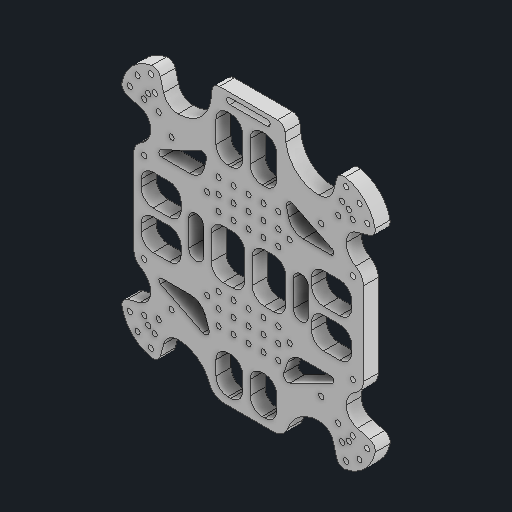
# Autodesk Inventor part: top
Saved by Autodesk Inventor 2023 (Build 270158000, 158)
## iProperties
Created: 2022-06-01
Part Number: top
Material: Generic
Document SubType Name: Modeling
Designer: vibhu
Density: 1 g/cm^3
Appearance: Default
Author: vibhu
Autodesk Inventor part; units mm, degrees
ref_plane "YZ Plane" through (0, 0, 0) normal (1, 0, 0) x (0, 1, 0)
ref_plane "XZ Plane" through (0, 0, 0) normal (0, 1, 0) x (-1, 0, 0)
ref_plane "Work Plane1" through (0, 0, 0) normal (0, 0, 1) x (1, 0, 0)
sketch "Sketch1" plane through (0, 0, 0) normal (0, 0, 1) x (1, 0, 0)
  arc A0 (58.1462, -72.4732) -> (48.4869, -65.0614) centre (48.4869, -75.0614) ccw projected
  line L0 (60.3557, -80.7192) -> (58.1462, -72.4732) projected
  arc A1 (60.3557, -80.7192) -> (66.1208, -84.3368) centre (65.1853, -79.4251) ccw projected
  arc A2 (66.1208, -84.3368) -> (86.0018, -64.4558) centre (61.4433, -59.7783) ccw projected
  arc A3 (86.0018, -64.4558) -> (82.3842, -58.6907) centre (81.0901, -63.5203) ccw projected
  line L1 (74.1382, -56.4812) -> (82.3842, -58.6907) projected
  arc A4 (66.7264, -46.8219) -> (74.1382, -56.4812) centre (76.7264, -46.8219) ccw projected
  circle A5 centre (61.4433, -59.7783) radius 1.75 projected
  circle A6 centre (68.5144, -66.8494) radius 1.75 projected
  circle A7 centre (64.0315, -69.4376) radius 1.75 projected
  circle A8 centre (71.1025, -62.3665) radius 1.75 projected
  circle A9 centre (80.7618, -64.9547) radius 1.75 projected
  circle A10 centre (75.5854, -73.9204) radius 1.75 projected
  circle A11 centre (66.6197, -79.0968) radius 1.75 projected
  line L2 (-55.2596, -72.4732) -> (-57.4691, -80.7192) projected
  arc A12 (-63.2342, -84.3368) -> (-57.4691, -80.7192) centre (-62.2987, -79.4251) ccw projected
  arc A13 (-83.1152, -64.4558) -> (-63.2342, -84.3368) centre (-58.5567, -59.7783) ccw projected
  arc A14 (-79.4976, -58.6907) -> (-83.1152, -64.4558) centre (-78.2035, -63.5203) ccw projected
  line L3 (-79.4976, -58.6907) -> (-71.2516, -56.4812) projected
  arc A15 (-71.2516, -56.4812) -> (-63.8398, -46.8219) centre (-73.8398, -46.8219) ccw projected
  arc A16 (-45.6003, -65.0614) -> (-55.2596, -72.4732) centre (-45.6003, -75.0614) ccw projected
  circle A17 centre (-61.1449, -69.4376) radius 1.75 projected
  circle A18 centre (-58.5567, -59.7783) radius 1.75 projected
  circle A19 centre (-65.6278, -66.8494) radius 1.75 projected
  circle A20 centre (-68.216, -62.3665) radius 1.75 projected
  circle A21 centre (-77.8752, -64.9547) radius 1.75 projected
  circle A22 centre (-72.6989, -73.9204) radius 1.75 projected
  circle A23 centre (-63.7331, -79.0968) radius 1.75 projected
  arc A24 (-63.8398, 47.2653) -> (-71.2516, 56.9246) centre (-73.8398, 47.2653) ccw projected
  line L4 (-71.2516, 56.9246) -> (-79.4976, 59.1341) projected
  arc A25 (-83.1152, 64.8992) -> (-79.4976, 59.1341) centre (-78.2035, 63.9637) ccw projected
  circle A26 centre (-77.8752, 65.3981) radius 1.75 projected
  arc A27 (-63.2342, 84.7802) -> (-83.1152, 64.8992) centre (-58.5567, 60.2217) ccw projected
  circle A28 centre (-68.216, 62.8099) radius 1.75 projected
  circle A29 centre (-58.5567, 60.2217) radius 1.75 projected
  circle A30 centre (-65.6278, 67.2928) radius 1.75 projected
  circle A31 centre (-61.1449, 69.881) radius 1.75 projected
  circle A32 centre (-72.6989, 74.3638) radius 1.75 projected
  circle A33 centre (-63.7331, 79.5402) radius 1.75 projected
  arc A34 (-57.4691, 81.1626) -> (-63.2342, 84.7802) centre (-62.2987, 79.8685) ccw projected
  line L5 (-57.4691, 81.1626) -> (-55.2596, 72.9166) projected
  arc A35 (-55.2596, 72.9166) -> (-45.6003, 65.5048) centre (-45.6003, 75.5048) ccw projected
  line L6 (13.9433, 88.2217) -> (-11.0567, 88.2217) projected
  arc A36 (13.9433, 88.2217) -> (13.9433, 92.2217) centre (13.9433, 90.2217) ccw projected
  line L7 (-11.0567, 92.2217) -> (13.9433, 92.2217) projected
  arc A37 (-11.0567, 92.2217) -> (-11.0567, 88.2217) centre (-11.0567, 90.2217) ccw projected
  line L8 (20.8532, 95.2217) -> (-17.9667, 95.2217) projected
  circle A38 centre (-18.5567, 80.2217) radius 1.75 construction
  circle A39 centre (-18.5567, 60.2217) radius 1.75 construction
  circle A40 centre (21.4433, 60.2217) radius 1.75 construction
  circle A41 centre (21.4433, 80.2217) radius 1.75 construction
  circle A42 centre (1.4433, 80.2217) radius 1.75 construction
  circle A43 centre (1.4433, 60.2217) radius 1.75 construction
  arc A44 (48.4869, 65.5048) -> (58.1462, 72.9166) centre (48.4869, 75.5048) ccw projected
  line L9 (58.1462, 72.9166) -> (60.3557, 81.1626) projected
  arc A45 (66.1208, 84.7802) -> (60.3557, 81.1626) centre (65.1853, 79.8685) ccw projected
  arc A46 (86.0018, 64.8992) -> (66.1208, 84.7802) centre (61.4433, 60.2217) ccw projected
  arc A47 (82.3842, 59.1341) -> (86.0018, 64.8992) centre (81.0901, 63.9637) ccw projected
  line L10 (82.3842, 59.1341) -> (74.1382, 56.9246) projected
  arc A48 (74.1382, 56.9246) -> (66.7264, 47.2653) centre (76.7264, 47.2653) ccw projected
  circle A49 centre (61.4433, 60.2217) radius 1.75 projected
  circle A50 centre (68.5144, 67.2928) radius 1.75 projected
  circle A51 centre (71.1025, 62.8099) radius 1.75 projected
  circle A52 centre (64.0315, 69.881) radius 1.75 projected
  circle A53 centre (66.6197, 79.5402) radius 1.75 projected
  circle A54 centre (75.5854, 74.3638) radius 1.75 projected
  circle A55 centre (80.7618, 65.3981) radius 1.75 projected
  circle A56 centre (71.4433, -19.7783) radius 1.75 construction
  circle A57 centre (51.4433, -19.7783) radius 1.75 construction
  circle A58 centre (51.4433, 20.2217) radius 1.75 construction
  circle A59 centre (61.4433, 20.2217) radius 1.75 construction
  circle A60 centre (-48.5567, 20.2217) radius 1.75 construction
  circle A61 centre (-68.5567, 20.2217) radius 1.75 construction
  circle A62 centre (-68.5567, -19.7783) radius 1.75 construction
  circle A63 centre (-48.5567, -19.7783) radius 1.75 construction
  circle A64 centre (-68.5567, 0.2217) radius 1.75 construction
  circle A65 centre (-48.5567, 0.2217) radius 1.75 construction
  circle A66 centre (-18.5567, -9.7783) radius 1.75 construction
  circle A67 centre (-18.5567, 10.2217) radius 1.75 construction
  circle A68 centre (21.4433, 10.2217) radius 1.75 construction
  circle A69 centre (21.4433, -9.7783) radius 1.75 construction
  circle A70 centre (1.4433, -9.7783) radius 1.75 construction
  circle A71 centre (1.4433, 10.2217) radius 1.75 construction
  circle A72 centre (-26.0567, -29.7783) radius 1.75 projected
  circle A73 centre (-26.0567, 30.2217) radius 1.75 projected
  circle A74 centre (28.9433, -29.7783) radius 1.75 projected
  circle A75 centre (28.9433, 30.2217) radius 1.75 projected
  circle A76 centre (-18.5567, -59.7783) radius 1.75 construction
  circle A77 centre (21.4433, -59.7783) radius 1.75 construction
  circle A78 centre (1.4433, -59.7783) radius 1.75 construction
  circle A79 centre (1.4433, -79.7783) radius 1.75 construction
  circle A80 centre (21.4433, -79.7783) radius 1.75 construction
  circle A81 centre (-18.5567, -79.7783) radius 1.75 construction
  arc A82 (-70.1082, 36.6881) -> (-63.8398, 47.2653) centre (-75.8979, 47.2653) ccw projected
  arc A83 (-70.1082, 36.6881) -> (-75.3067, 27.9162) centre (-65.3067, 27.9162) ccw projected
  line L11 (-75.3067, 27.9162) -> (-75.3067, -27.4729) projected
  arc A84 (-75.3067, -27.4729) -> (-70.1082, -36.2447) centre (-65.3067, -27.4729) ccw projected
  arc A85 (-63.8398, -46.8219) -> (-70.1082, -36.2447) centre (-75.8979, -46.8219) ccw projected
  arc A86 (-24.7861, -79.8307) -> (-45.6003, -65.0614) centre (-45.6003, -87.1128) ccw projected
  arc A87 (-24.7861, -79.8307) -> (-15.3471, -86.5283) centre (-15.3471, -76.5283) ccw projected
  line L12 (-15.3471, -86.5283) -> (18.2337, -86.5283) projected
  arc A88 (18.2337, -86.5283) -> (27.6726, -79.8307) centre (18.2337, -76.5283) ccw projected
  arc A89 (48.4869, -65.0614) -> (27.6726, -79.8307) centre (48.4869, -87.1128) ccw projected
  arc A90 (72.9948, -36.2447) -> (66.7264, -46.8219) centre (78.7845, -46.8219) ccw projected
  arc A91 (72.9948, -36.2447) -> (78.1933, -27.4729) centre (68.1933, -27.4729) ccw projected
  line L13 (78.1933, -27.4729) -> (78.1933, 27.9162) projected
  arc A92 (78.1933, 27.9162) -> (72.9948, 36.6881) centre (68.1933, 27.9162) ccw projected
  arc A93 (66.7264, 47.2653) -> (72.9948, 36.6881) centre (78.7845, 47.2653) ccw projected
  arc A94 (26.4433, 85.2217) -> (48.4869, 65.5048) centre (48.4869, 87.6857) ccw projected
  line L14 (26.4433, 85.2217) -> (25.8223, 90.7771) projected
  arc A95 (25.8223, 90.7771) -> (20.8532, 95.2217) centre (20.8532, 90.2217) ccw projected
  arc A96 (-17.9667, 95.2217) -> (-22.9357, 90.7771) centre (-17.9667, 90.2217) ccw projected
  line L15 (-22.9357, 90.7771) -> (-23.5567, 85.2217) projected
  arc A97 (-45.6003, 65.5048) -> (-23.5567, 85.2217) centre (-45.6003, 87.6857) ccw projected
  circle A98 centre (-68.3067, 30.2217) radius 1.75 projected
  circle A99 centre (-68.3067, -29.7783) radius 1.75 projected
  circle A100 centre (71.1933, -29.7783) radius 1.75 projected
  circle A101 centre (71.1933, 30.2217) radius 1.75 projected
  arc A102 (-28.5567, 9.0414) -> (-38.5567, 9.0414) centre (-33.5567, 9.0414) ccw projected
  line L16 (-38.5567, -8.598) -> (-38.5567, 9.0414) projected
  arc A103 (-38.5567, -8.598) -> (-28.5567, -8.598) centre (-33.5567, -8.598) ccw projected
  line L17 (-28.5567, 9.0414) -> (-28.5567, -8.598) projected
  line L18 (31.4433, -8.598) -> (31.4433, 9.0414) projected
  arc A104 (41.4433, 9.0414) -> (31.4433, 9.0414) centre (36.4433, 9.0414) ccw projected
  line L19 (41.4433, 9.0414) -> (41.4433, -8.598) projected
  arc A105 (31.4433, -8.598) -> (41.4433, -8.598) centre (36.4433, -8.598) ccw projected
  line L20 (1.4433, 104.693) -> (1.4433, -135.8367) construction
  circle A106 centre (-18.5567, 22.451) radius 1.75
  line L21 (1.4433, -94.5531) -> (25.8223, -94.5531) construction
  circle A107 centre (-18.5567, 32.451) radius 1.75
  circle A108 centre (-18.5567, 42.451) radius 1.75
  circle A109 centre (-8.5567, 22.451) radius 1.75
  circle A110 centre (-8.5567, 32.451) radius 1.75
  circle A111 centre (-8.5567, 42.451) radius 1.75
  circle A112 centre (1.4433, 22.451) radius 1.75
  circle A113 centre (1.4433, 32.451) radius 1.75
  circle A114 centre (1.4433, 42.451) radius 1.75
  circle A115 centre (11.4433, 22.451) radius 1.75
  circle A116 centre (11.4433, 32.451) radius 1.75
  circle A117 centre (11.4433, 42.451) radius 1.75
  circle A118 centre (21.4433, 22.451) radius 1.75
  circle A119 centre (21.4433, 32.451) radius 1.75
  circle A120 centre (21.4433, 42.451) radius 1.75
  line L22 (-3.5567, 35.8119) -> (-34.2609, 35.8119) construction
  line L23 (-36.5279, 29.0902) -> (-8, 29.0902) construction
  line L24 (-15.4957, 35.8119) -> (-15.4957, 29.0902) construction
  circle A121 centre (-18.5567, -23.7293) radius 1.75
  circle A122 centre (-18.5567, -33.7293) radius 1.75
  circle A123 centre (-18.5567, -43.7293) radius 1.75
  circle A124 centre (-8.5567, -23.7293) radius 1.75
  circle A125 centre (-8.5567, -33.7293) radius 1.75
  circle A126 centre (-8.5567, -43.7293) radius 1.75
  circle A127 centre (1.4433, -23.7293) radius 1.75
  circle A128 centre (1.4433, -33.7293) radius 1.75
  circle A129 centre (1.4433, -43.7293) radius 1.75
  circle A130 centre (11.4433, -23.7293) radius 1.75
  circle A131 centre (11.4433, -33.7293) radius 1.75
  circle A132 centre (11.4433, -43.7293) radius 1.75
  circle A133 centre (21.4433, -23.7293) radius 1.75
  circle A134 centre (21.4433, -33.7293) radius 1.75
  circle A135 centre (21.4433, -43.7293) radius 1.75
  line L25 (-6.5567, -30.3685) -> (-35.0846, -30.3685) construction
  line L26 (-35.7042, -37.0902) -> (-5, -37.0902) construction
  line L27 (-15.1289, -30.3685) -> (-15.1289, -37.0902) construction
  point P0 (0, 0)
  point P1 (-75.3067, 0.2217)
  point P2 (-15.4957, 32.451)
  point P3 (-15.1289, -33.7293)
  dimension "d6" = 3.5
  dimension "d9" = 10
  dimension "d12" = 10
  dimension "d17" = 10
  dimension "d20" = 10
  constraints: 30 centre point, 12 end point, 6 point on line, 5 horizontal, 3 midpoint, 3 vertical, 2 horizontal alignment, 2 perpendicular, 2 vertical alignment, 1 equal radius, 60 other
  measures "d6" diameter of A106
  measures "d9" distance of A106.centre A107.centre
  measures "d12" distance of A106.centre A109.centre
  measures "d17" distance of A121.centre A122.centre
  measures "d20" distance of A121.centre A124.centre
extrude "Extrusion1" add sketch "Sketch1" along normal blind 10
sketch "Sketch2" plane through (0, 0, 10) normal (0, 0, 1) x (1, 0, 0)
  circle A0 centre (-18.5567, -59.7783) radius 1.75 construction
  circle A1 centre (-18.5567, -79.7783) radius 1.75 construction
  circle A2 centre (21.4433, -79.7783) radius 1.75 construction
  circle A3 centre (21.4433, -59.7783) radius 1.75 construction
  circle A4 centre (51.4433, -19.7783) radius 1.75 construction
  circle A5 centre (71.4433, -19.7783) radius 1.75 construction
  circle A6 centre (51.4433, 20.2217) radius 1.75 construction
  circle A7 centre (-68.5567, 20.2217) radius 1.75 construction
  circle A8 centre (-48.5567, 20.2217) radius 1.75 construction
  circle A9 centre (-68.5567, -19.7783) radius 1.75 construction
  circle A10 centre (-48.5567, -19.7783) radius 1.75 construction
  circle A11 centre (-18.5567, 60.2217) radius 1.75 construction
  circle A12 centre (21.4433, 60.2217) radius 1.75 construction
  circle A13 centre (21.4433, 80.2217) radius 1.75 construction
  circle A14 centre (-18.5567, 80.2217) radius 1.75 construction
  circle A15 centre (-18.5567, -9.7783) radius 1.75 construction
  circle A16 centre (21.4433, -9.7783) radius 1.75 construction
  circle A17 centre (21.4433, 10.2217) radius 1.75 construction
  circle A18 centre (-18.5567, 10.2217) radius 1.75 construction
  line L0 (-70.3067, 23.4717) -> (-43.5567, 23.4717)
  line L1 (-43.5567, 23.4717) -> (-43.5567, -23.0283)
  line L2 (-43.5567, -23.0283) -> (-70.3067, -23.0283)
  line L3 (-70.3067, -23.0283) -> (-70.3067, 23.4717)
  line L4 (-75.3067, 27.9162) -> (-75.3067, -27.4729) projected
  circle A19 centre (-68.3067, 30.2217) radius 1.75 projected
  line L5 (-38.5567, -8.598) -> (-38.5567, 9.0414) projected
  line L6 (-70.3067, 2.7217) -> (-43.5567, 2.7217)
  line L7 (-43.5567, 2.7217) -> (-43.5567, -2.2783)
  line L8 (-43.5567, -2.2783) -> (-70.3067, -2.2783)
  line L9 (-70.3067, -2.2783) -> (-70.3067, 2.7217)
  line L10 (-23.5567, 15.701) -> (26.4433, 15.701)
  line L11 (26.4433, 15.701) -> (26.4433, -16.9793)
  line L12 (26.4433, -16.9793) -> (-23.5567, -16.9793)
  line L13 (-23.5567, -16.9793) -> (-23.5567, 15.701)
  line L14 (-28.5567, 9.0414) -> (-28.5567, -8.598) projected
  line L15 (31.4433, -8.598) -> (31.4433, 9.0414) projected
  circle A20 centre (-18.5567, 22.451) radius 1.75 construction
  circle A21 centre (-18.5567, -23.7293) radius 1.75 construction
  line L16 (-1.0567, 15.701) -> (3.9433, 15.701)
  line L17 (3.9433, 15.701) -> (3.9433, -16.9793)
  line L18 (3.9433, -16.9793) -> (-1.0567, -16.9793)
  line L19 (-1.0567, -16.9793) -> (-1.0567, 15.701)
  line L20 (0, 120.2032) -> (0, -113.5378) construction
  line L21 (-20.3067, 83.2217) -> (20.3067, 83.2217)
  line L22 (20.3067, 83.2217) -> (20.3067, 52.451)
  line L23 (20.3067, 52.451) -> (-20.3067, 52.451)
  line L24 (-20.3067, 52.451) -> (-20.3067, 83.2217)
  line L25 (-2.5, 83.2217) -> (2.5, 83.2217)
  line L26 (2.5, 83.2217) -> (2.5, 52.451)
  line L27 (2.5, 52.451) -> (-2.5, 52.451)
  line L28 (-2.5, 52.451) -> (-2.5, 83.2217)
  line L29 (13.9433, 88.2217) -> (-11.0567, 88.2217) projected
  circle A22 centre (-18.5567, 42.451) radius 1.75 projected
  line L30 (0, 0) -> (110.9609, 0) construction
  circle A23 centre (68.5567, 20.2217) radius 1.75 construction
  circle A24 centre (48.5567, 20.2217) radius 1.75 construction
  circle A25 centre (68.5567, -19.7783) radius 1.75 construction
  circle A26 centre (48.5567, -19.7783) radius 1.75 construction
  line L31 (70.3067, 23.4717) -> (43.5567, 23.4717)
  line L32 (43.5567, 23.4717) -> (43.5567, -23.0283)
  line L33 (43.5567, -23.0283) -> (70.3067, -23.0283)
  line L34 (70.3067, -23.0283) -> (70.3067, 23.4717)
  line L35 (70.3067, 2.7217) -> (43.5567, 2.7217)
  line L36 (43.5567, 2.7217) -> (43.5567, -2.2783)
  line L37 (43.5567, -2.2783) -> (70.3067, -2.2783)
  line L38 (70.3067, -2.2783) -> (70.3067, 2.7217)
  line L39 (-20.3067, -56.0283) -> (20.3067, -56.0283)
  line L40 (20.3067, -56.0283) -> (20.3067, -81.5283)
  line L41 (20.3067, -81.5283) -> (-20.3067, -81.5283)
  line L42 (-20.3067, -81.5283) -> (-20.3067, -56.0283)
  line L43 (-2.5, -56.0283) -> (2.5, -56.0283)
  line L44 (2.5, -56.0283) -> (2.5, -81.5283)
  line L45 (2.5, -81.5283) -> (-2.5, -81.5283)
  line L46 (-2.5, -81.5283) -> (-2.5, -56.0283)
  line L47 (-15.3471, -86.5283) -> (18.2337, -86.5283) projected
  point P0 (-38.5567, 0.2217)
  point P1 (-43.5567, 0.2217)
  point P2 (-43.5567, 0.2217)
  point P3 (1.4433, 15.701)
  point P4 (1.4433, 15.701)
  point P5 (0, 83.2217)
  point P6 (0, 83.2217)
  point P7 (43.5567, 0.2217)
  point P8 (43.5567, 0.2217)
  point P9 (0, -56.0283)
  point P10 (0, -56.0283)
  point P11 (-43.5567, -2.2783)
  point P12 (-70.3067, -2.2783)
  point P13 (-70.3067, 2.7217)
  point P14 (-43.5567, 2.7217)
  point P15 (-1.0567, 15.701)
  point P16 (43.5567, 2.7217)
  point P17 (70.3067, 2.7217)
  point P18 (70.3067, -2.2783)
  point P19 (43.5567, -2.2783)
  dimension "d25" = 5
  dimension "d27" = 5
  dimension "d28" = 5
  dimension "d29" = 5
  dimension "d30" = 5
  dimension "d31" = 5
  dimension "d33" = 5
  dimension "d34" = 5
  dimension "d35" = 5
  dimension "d36" = 5
  dimension "d37" = 10
  dimension "d38" = 5
  dimension "d40" = 5
  dimension "d41" = 5
  dimension "d42" = 2
  constraints: 84 end point, 16 parallel, 14 symmetric about line, 9 horizontal, 9 midpoint, 8 collinear, 8 perpendicular, 4 centre point, 4 coincident, 3 point on line, 2 tangent, 1 horizontal alignment, 1 vertical, 4 other
  measures "d25" distance between parallel lines of L4 L3
  measures "d27" distance edge to line of A19 L0
  measures "d28" distance between parallel lines of L5 L1
  measures "d29" distance between parallel lines of L8 L6
  measures "d30" distance between parallel lines of L13 L14
  measures "d31" distance between parallel lines of L15 L11
  measures "d33" distance edge to line of A20 L10
  measures "d34" distance edge to line of A21 L12
  measures "d35" distance between parallel lines of L17 L19
  measures "d36" distance between parallel lines of L21 L29
  measures "d37" distance from line of A22.centre L23
  measures "d38" distance between parallel lines of L26 L28
  measures "d40" distance between parallel lines of L44 L46
  measures "d41" distance between parallel lines of L41 L47
  measures "d42" distance edge to line of A0 L39
extrude "Extrusion2" cut sketch "Sketch2" against normal up to surface (10 mm away) contours L0 L1 L6 L3 | L8 L1 L2 L3 | L10 L19 L12 L13 | L10 L11 L12 L17 | L21 L28 L23 L24 | L21 L22 L23 L26 | L34 L35 L32 L31 | L34 L33 L32 L37 | L39 L46 L41 L42 | L39 L40 L41 L44
fillet "Fillet1" radius 8 40 edges at (-43.5567, -23.0283, 5) (-43.5567, -2.2783, 5) (-43.5567, 23.4717, 5) (-43.5567, 2.7217, 5) (-70.3067, 23.4717, 5) (-70.3067, 2.7217, 5) (-70.3067, -2.2783, 5) (-70.3067, -23.0283, 5) (-20.3067, -56.0283, 5) (-2.5, -56.0283, 5) (2.5, -56.0283, 5) (20.3067, -56.0283, 5) (20.3067, -81.5283, 5) (2.5, -81.5283, 5) (-2.5, -81.5283, 5) (-20.3067, -81.5283, 5) (-1.0567, 15.701, 5) (-23.5567, 15.701, 5) (-23.5567, -16.9793, 5) (-1.0567, -16.9793, 5) (3.9433, -16.9793, 5) (3.9433, 15.701, 5) (26.4433, 15.701, 5) (26.4433, -16.9793, 5) (70.3067, 23.4717, 5) (70.3067, 2.7217, 5) (70.3067, -2.2783, 5) (70.3067, -23.0283, 5) (43.5567, -23.0283, 5) (43.5567, -2.2783, 5) (43.5567, 2.7217, 5) (43.5567, 23.4717, 5) (-2.5, 52.451, 5) (2.5, 52.451, 5) (2.5, 83.2217, 5) (-2.5, 83.2217, 5) (-20.3067, 83.2217, 5) (-20.3067, 52.451, 5) (20.3067, 83.2217, 5) (20.3067, 52.451, 5)
sketch "Sketch3" plane through (0, 0, 10) normal (0, 0, 1) x (1, 0, 0)
  line L0 (-50, 50) -> (50, 50) construction
  line L1 (50, 50) -> (50, -50) construction
  line L2 (50, -50) -> (-50, -50) construction
  line L3 (-50, -50) -> (-50, 50) construction
  line L4 (-50, 50) -> (50, -50) construction
  line L5 (50, 50) -> (-50, -50) construction
  circle A0 centre (-50, 50) radius 1.75
  circle A1 centre (50, 50) radius 1.75
  circle A2 centre (50, -50) radius 1.75
  circle A3 centre (-50, -50) radius 1.75
  point P0 (0, 0)
  dimension "d46" = 100
  dimension "d47" = 100
  dimension "d48" = 3.5
  constraints: 12 end point, 4 centre point, 4 coincident, 3 equal radius, 2 midpoint, 2 parallel, 1 horizontal, 1 perpendicular
  measures "d46" distance of L1.end L2.end
  measures "d47" distance of L0.end L1.end
  measures "d48" diameter of A0
extrude "Extrusion3" cut sketch "Sketch3" against normal up to surface (10 mm away)
sketch "Sketch4" plane through (0, 0, 0) normal (0, 0, -1) x (-1, 0, 0)
  circle A0 centre (-21.4433, 42.451) radius 1.75 construction
  circle A1 centre (-21.4433, 42.451) radius 3.25
  circle A2 centre (-21.4433, -23.7293) radius 1.75 construction
  circle A3 centre (-21.4433, -23.7293) radius 3.25
  line L0 (0, 0) -> (22.8644, 0) construction
  line L1 (22.8644, 0) -> (0, 0)
  line L2 (0, 16.9905) -> (0, 0) construction
  circle A4 centre (-11.4433, -23.7293) radius 3.25
  circle A5 centre (-1.4433, -23.7293) radius 3.25
  circle A6 centre (8.5567, -23.7293) radius 3.25
  circle A7 centre (18.5567, -23.7293) radius 3.25
  circle A8 centre (-21.4433, -33.7293) radius 3.25
  circle A9 centre (-11.4433, -33.7293) radius 3.25
  circle A10 centre (-1.4433, -33.7293) radius 3.25
  circle A11 centre (8.5567, -33.7293) radius 3.25
  circle A12 centre (18.5567, -33.7293) radius 3.25
  circle A13 centre (-21.4433, -43.7293) radius 3.25
  circle A14 centre (-11.4433, -43.7293) radius 3.25
  circle A15 centre (-1.4433, -43.7293) radius 3.25
  circle A16 centre (8.5567, -43.7293) radius 3.25
  circle A17 centre (18.5567, -43.7293) radius 3.25
  circle A18 centre (-11.4433, 42.451) radius 3.25
  circle A19 centre (-1.4433, 42.451) radius 3.25
  circle A20 centre (8.5567, 42.451) radius 3.25
  circle A21 centre (18.5567, 42.451) radius 3.25
  circle A22 centre (-21.4433, 32.451) radius 3.25
  circle A23 centre (-11.4433, 32.451) radius 3.25
  circle A24 centre (-1.4433, 32.451) radius 3.25
  circle A25 centre (8.5567, 32.451) radius 3.25
  circle A26 centre (18.5567, 32.451) radius 3.25
  circle A27 centre (-21.4433, 22.451) radius 3.25
  circle A28 centre (-11.4433, 22.451) radius 3.25
  circle A29 centre (-1.4433, 22.451) radius 3.25
  circle A30 centre (8.5567, 22.451) radius 3.25
  circle A31 centre (18.5567, 22.451) radius 3.25
  dimension "d51" = 6.5
  dimension "d52" = 6.5
  dimension "d60" = 10
  dimension "d63" = 10
  dimension "d68" = 10
  dimension "d71" = 10
  constraints: 30 centre point, 6 end point, 3 horizontal, 2 coincident, 2 vertical, 1 collinear, 1 perpendicular, 56 other
  measures "d51" diameter of A1
  measures "d52" diameter of A3
  measures "d60" distance of A3.centre A4.centre
  measures "d63" distance of A3.centre A8.centre
  measures "d68" distance of A1.centre A18.centre
  measures "d71" distance of A1.centre A22.centre
extrude "Extrusion4" cut sketch "Sketch4" against normal blind 3
sketch "Sketch5" plane through (0, 0, 10) normal (0, 0, 1) x (1, 0, 0)
  line L0 (-65, 35) -> (-30, 35)
  line L1 (-30, 35) -> (-25.3067, 54.7437)
  line L2 (-25.3067, 54.7437) -> (-65, 35)
  line L3 (25.3067, 54.7437) -> (30, 35)
  line L4 (30, 35) -> (65, 35)
  line L5 (65, 35) -> (25.3067, 54.7437)
  line L6 (30, -35) -> (65, -35)
  line L7 (65, -35) -> (22.4502, -56.1645)
  line L8 (22.4502, -56.1645) -> (30, -35)
  line L9 (-65, -35) -> (-30, -35)
  line L10 (-30, -35) -> (-22.4502, -56.1645)
  line L11 (-22.4502, -56.1645) -> (-65, -35)
  line L12 (-30, -35) -> (30, -35) construction
  line L13 (30, -35) -> (30, 35) construction
  line L14 (30, 35) -> (-30, 35) construction
  line L15 (-30, 35) -> (-30, -35) construction
  line L16 (-30, -35) -> (30, 35) construction
  line L17 (30, -35) -> (-30, 35) construction
  line L18 (-22.4502, -56.1645) -> (22.4502, -56.1645) construction
  line L19 (-25.3067, 54.7437) -> (25.3067, 54.7437) construction
  line L20 (-20.3067, 60.451) -> (-20.3067, 75.2217) projected
  circle A0 centre (-50, 50) radius 1.75 projected
  circle A1 centre (-50, -50) radius 1.75 projected
  arc A2 (-12.3067, -56.0283) -> (-20.3067, -64.0283) centre (-12.3067, -64.0283) ccw projected
  point P0 (0, 0)
  point P1 (0, -35)
  point P2 (0, -56.1645)
  point P3 (0, 54.7437)
  point P4 (0, 35)
  point P5 (-17.9636, -58.3714)
  dimension "d76" = 70
  dimension "d77" = 5
  dimension "d78" = 5
  dimension "d79" = 5
  dimension "d80" = 35
  dimension "d81" = 60
  dimension "d82" = 5
  constraints: 41 end point, 6 midpoint, 5 vertical alignment, 4 horizontal, 3 equal length, 2 collinear, 2 horizontal alignment, 2 point on line, 1 perpendicular, 1 point on circle
  measures "d76" distance of L0.end L12.start
  measures "d77" distance from line of L20 L1.end
  measures "d78" distance edge to line of A0 L2
  measures "d79" distance edge to line of A1 L11
  measures "d80" distance of L0.start L0.end
  measures "d81" distance of L3.end L0.end
  measures "d82" distance of point (-17.964, -58.371) L10.end
extrude "Extrusion5" cut sketch "Sketch5" against normal up to surface (10 mm away) contours L2 L1 L0 | L5 L4 L3 | L6 L7 L8 | L9 L10 L11
fillet "Fillet2" radius 3 4 edges at (25.3067, 54.7437, 5) (-25.3067, 54.7437, 5) (-22.4502, -56.1645, 5) (22.4502, -56.1645, 5)
fillet "Fillet3" radius 10 4 edges at (30, -35, 5) (30, 35, 5) (-30, 35, 5) (-30, -35, 5)
fillet "Fillet4" radius 2 4 edges at (65, 35, 5) (65, -35, 5) (-65, -35, 5) (-65, 35, 5)
body "Solid1"
